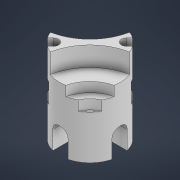
# Autodesk Inventor part: mount-stem
Saved by Autodesk Inventor 2021 (Build 250183000, 183)
## iProperties
Created: 2024-05-22
Part Number: mount-stem
Material: Generic
Document SubType Name: Modeling
Designer: loren
Density: 1 g/cm^3
Appearance: Default
Author: loren
Autodesk Inventor part; units mm, degrees
ref_plane "YZ Plane" through (0, 0, 0) normal (1, 0, 0) x (0, 1, 0)
ref_plane "XZ Plane" through (0, 0, 0) normal (0, 1, 0) x (-1, 0, 0)
sketch "Sketch1" plane through (0, 0, 0) normal (0, 1, 0) x (-1, 0, 0)
  circle A0 centre (0, 0) radius 12.5
  dimension "d0" = 25
  constraints: 1 centre point, 1 coincident
  measures "d0" diameter of A0
extrude "Extrusion1" add sketch "Sketch1" along normal blind 19 and the other way blind 15
sketch "Sketch2" plane through (0, 0, 0) normal (0, 0, 1) x (1, 0, 0)
  line L0 (-5.25, -15) -> (-5.25, -7.5)
  arc A0 (5.25, -7.5) -> (-5.25, -7.5) centre (0, -7.5) ccw
  line L1 (5.25, -7.5) -> (5.25, -15)
  line L2 (5.25, -15) -> (-5.25, -15)
  line L3 (-3.1, -15) -> (-3.1, -7.5)
  arc A1 (3.1, -7.5) -> (-3.1, -7.5) centre (0, -7.5) ccw
  line L4 (3.1, -7.5) -> (3.1, -15)
  line L5 (0, 0) -> (0, -15) construction
  line L6 (-12.5, -15) -> (12.5, -15) projected
  point P0 (0, -7.5)
  dimension "d5" = 10.5
  dimension "d6" = 6.2
  constraints: 12 end point, 4 point on circle, 4 tangent, 3 point on line, 2 centre point, 2 midpoint, 2 perpendicular, 2 vertical, 1 coincident, 1 concentric, 1 parallel
  measures "d5" distance between parallel lines of L1 L0
  measures "d6" distance between parallel lines of L4 L3
extrude "Extrusion2" cut sketch "Sketch2" along normal mid plane 10.5
extrude "Extrusion3" cut sketch "Sketch2" against normal through all both and the other way through all contours L3 A1 L4 L2
pattern_circular "Circular Pattern1" count 2 over 90 about axis through (0, -10, 0) along (0, 1, 0) of "Extrusion2", "Extrusion3"
ref_plane "Work Plane1" through (0, 7.5, 0) normal (0, 1, 0) x (1, 0, 0)
sketch "Sketch3" plane through (0, 7.5, 0) normal (0, 1, 0) x (1, 0, 0)
  line L0 (7.2283, 10.1981) -> (6.0151, 8.9849)
  arc A0 (6.0151, 8.9849) -> (8.9849, 6.0151) centre (7.5, 7.5) ccw
  line L1 (8.9849, 6.0151) -> (10.1981, 7.2283)
  arc A1 (12.1095, 3.1) -> (3.1, 12.1095) centre (0, 0) ccw projected
  line L2 (0, 0) -> (7.5, 7.5) construction
  line L3 (-17.671, 0) -> (18.5127, 0) projected
  line L4 (5.9188, 11.0099) -> (4.9544, 10.0456)
  arc A2 (4.9544, 10.0456) -> (10.0456, 4.9544) centre (7.5, 7.5) ccw
  line L5 (10.0456, 4.9544) -> (11.0099, 5.9188)
  dimension "d15" = 4.2
  dimension "d16" = 7.5
  dimension "d17" = 45
  dimension "d18" = 7.2
  constraints: 10 end point, 8 point on circle, 4 parallel, 4 tangent, 2 centre point, 1 coincident
  measures "d15" distance between parallel lines of L1 L0
  measures "d16" horizontal distance of L2.end L2.start
  measures "d17" angle of L2 L3
  measures "d18" distance between parallel lines of L5 L4
extrude "Extrusion4" cut sketch "Sketch3" along normal through all both and the other way through all contours A1 L1 A0 L0
extrude "Extrusion5" cut sketch "Sketch3" against normal blind 8
pattern_circular "Circular Pattern2" count 2 over 360 about axis through (0, -10, 0) along (0, 1, 0) of "Extrusion4", "Extrusion5"
sketch "Sketch4" plane through (0, 19, 0) normal (0, 1, 0) x (1, 0, 0)
  circle A0 centre (-15.5, 15.5) radius 20.5
  line L0 (-15.5, 15.5) -> (15.5, 15.5) construction
  line L1 (15.5, 15.5) -> (15.5, -15.5) construction
  line L2 (15.5, -15.5) -> (-15.5, -15.5) construction
  line L3 (-15.5, -15.5) -> (-15.5, 15.5) construction
  circle A1 centre (-15.5, 15.5) radius 13.5
  circle A2 centre (-15.5, 15.5) radius 10.5
  point P0 (0, 0)
  point P1 (15.5, 0)
  point P2 (0, 15.5)
  dimension "d27" = 41
  dimension "d28" = 31
  dimension "d31" = 27
  dimension "d32" = 21
  constraints: 8 end point, 3 centre point, 2 coincident, 2 midpoint, 2 parallel, 2 perpendicular, 1 horizontal, 1 horizontal alignment, 1 vertical alignment
  measures "d27" diameter of A0
  measures "d28" distance of L0.start L0.end
  measures "d31" diameter of A1
  measures "d32" diameter of A2
extrude "Extrusion6" cut sketch "Sketch4" against normal blind 8 contours A0 | A1 | A2
extrude "Extrusion7" cut sketch "Sketch4" against normal blind 12 contours A1 | A2
extrude "Extrusion8" cut sketch "Sketch4" against normal blind 16 contours A2
pattern_circular "Circular Pattern3" count 2 over 360 about axis through (0, -10, 0) along (0, 1, 0) of "Extrusion7", "Extrusion6", "Extrusion8"
body "Solid1"
